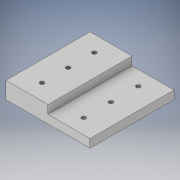
# Autodesk Inventor part: screwbase
Saved by Autodesk Inventor 2019 (Build 230136000, 136)
## iProperties
Created: 2018-12-19
Part Number: screwbase
Material: Generic
Document SubType Name: Modeling
Designer: assman
Density: 1 g/cm^3
Appearance: Default
Author: assman
Autodesk Inventor part; units mm, degrees
ref_plane "YZ Plane" through (0, 0, 0) normal (1, 0, 0) x (0, 1, 0)
ref_plane "XZ Plane" through (0, 0, 0) normal (0, 1, 0) x (-1, 0, 0)
ref_plane "XY Plane" through (0, 0, 0) normal (0, 0, 1) x (1, 0, 0)
sketch "Sketch1" plane through (0, 0, 0) normal (0, 1, 0) x (-1, 0, 0)
  line L0 (25, 25) -> (-25, 25)
  line L1 (-25, 25) -> (-25, -25)
  line L2 (-25, -25) -> (25, -25)
  line L3 (25, -25) -> (25, 25)
  line L4 (35, 0) -> (-35, 0) projected
  line L5 (0, -35) -> (0, 35) projected
  point P0 (0, 0)
  dimension "d0" = 50
  dimension "d1" = 50
  constraints: 8 end point, 2 parallel, 1 horizontal, 1 perpendicular, 2 other
  measures "d0" distance of L0.start L0.end
  measures "d1" distance of L2.end L0.start
extrude "Extrusion1" add sketch "Sketch1" along normal blind 10
sketch "Sketch2" plane through (0, 10, 0) normal (0, 1, 0) x (1, 0, 0)
  line L0 (-25, -25) -> (25, -25) projected
  line L1 (25, -25) -> (25, 25) projected
  line L2 (0, -25) -> (25, -25)
  line L3 (25, -25) -> (25, 25)
  line L4 (25, 25) -> (0, 25)
  line L5 (0, 25) -> (0, -25)
  point P0 (0, 0)
  constraints: 8 end point, 2 parallel, 1 horizontal, 1 midpoint, 1 perpendicular
extrude "Extrusion2" cut sketch "Sketch2" against normal blind 5
sketch "Sketch3" plane through (0, 10, 0) normal (0, 1, 0) x (1, 0, 0)
  line L0 (-12.9579, -25.0914) -> (-12.9579, 25) construction
  line L1 (25, 25) -> (-25, 25) construction
  line L2 (12.5042, -25.0914) -> (12.5042, 25) construction
  line L3 (-35, 0) -> (35, 0) construction
  point P0 (0, 0)
  point P1 (-12.9579, -0.0457)
  point P2 (-12.9579, -15.5571)
  point P3 (-12.9579, 15.5571)
  point P4 (12.5042, -16.2302)
  point P5 (12.5042, -0.0457)
  point P6 (12.5042, 16.2302)
  constraints: 6 point on line, 4 end point, 2 midpoint, 2 symmetric about line, 1 parallel, 1 vertical
hole "Hole1" at (-12.9579, 10, 0.0457) at (-12.9579, 10, -15.5571) at (12.5042, 10, 16.2302) at (12.5042, 10, 0.0457) at (12.5042, 10, -16.2302) at (-12.9579, 10, 15.5571) direction (0, -1, 0) diameter 2.459 depth 10 thread size "M3x0.5" class "6H" standard "ISO Metric profile"
equation "\"d1\" = d0"
body "Solid1"
